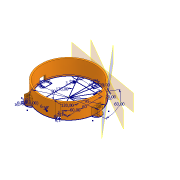
# Autodesk Inventor part: TopPart
Saved by Autodesk Inventor 2020.3 (Build 243373000, 373)
## iProperties
Created: 2021-08-28
Part Number: TopPart
Material: Generic
Document SubType Name: Modeling
Designer: Yusuf
Mass: 20.7363 g
Surface Area: 175.802 cm^2
Volume: 20.7363 cm^3
Density: 1 g/cm^3
Appearance: Orange
Author: Yusuf
Autodesk Inventor part; units mm, degrees
ref_plane "YZ Plane" through (0, 0, 0) normal (1, 0, 0) x (0, 1, 0)
ref_plane "XZ Plane" through (0, 0, 0) normal (0, 1, 0) x (-1, 0, 0)
ref_plane "XY Plane" through (0, 0, 0) normal (0, 0, 1) x (1, 0, 0)
sketch "Sketch1" plane through (0, 0, 0) normal (0, 1, 0) x (-1, 0, 0)
  circle A0 centre (0, 0) radius 47.5
  line L0 (0, 0) -> (23.75, 41.1362)
  line L1 (0, 0) -> (23.75, -41.1362)
  line L2 (0, 0) -> (-47.5, 0)
  circle A1 centre (23.75, 41.1362) radius 8
  circle A2 centre (25.75, 44.6003) radius 1.7
  circle A3 centre (25.75, 44.6003) radius 3.25
  line L3 (23.75, 41.1362) -> (27.75, 48.0644)
  arc A4 (30.4398, 45.5233) -> (30.3168, 36.567) centre (39.3185, 40.9223) ccw
  arc A5 (29.9181, 44.333) -> (29.4758, 46.7233) centre (27.662, 45.1516) ccw
  arc A6 (16.5096, 44.5386) -> (24.2044, 49.1233) centre (15.7805, 54.512) ccw
  arc A7 (25.7257, 48.8884) -> (23.4345, 48.0763) centre (25.2714, 46.5318) ccw
  circle A8 centre (-47.5, 0) radius 8
  arc A9 (-54.6442, 3.6) -> (-46.8263, 7.9716) centre (-55.099, 13.5897) ccw
  circle A10 centre (-51.5, 0) radius 3.25
  circle A11 centre (-51.5, 0) radius 1.7
  line L4 (-47.5, 0) -> (-55.5, 0)
  arc A12 (-53.3526, 3.7433) -> (-55.2014, 2.1651) centre (-52.9334, 1.3802) ccw
  arc A13 (-55.2014, -2.1651) -> (-53.3526, -3.7433) centre (-52.9334, -1.3802) ccw
  arc A14 (-46.8263, -7.9716) -> (-54.6442, -3.6) centre (-55.099, -13.5897) ccw
  circle A15 centre (23.75, -41.1362) radius 8
  arc A16 (24.2044, -49.1233) -> (16.5096, -44.5386) centre (15.7805, -54.512) ccw
  circle A17 centre (25.75, -44.6003) radius 3.25
  circle A18 centre (25.75, -44.6003) radius 1.7
  line L5 (23.75, -41.1362) -> (27.75, -48.0644)
  arc A19 (23.4345, -48.0763) -> (25.7257, -48.8884) centre (25.2714, -46.5318) ccw
  arc A20 (29.4758, -46.7233) -> (29.9181, -44.333) centre (27.662, -45.1516) ccw
  arc A21 (30.3168, -36.567) -> (30.4398, -45.5233) centre (39.3185, -40.9223) ccw
  line L6 (47.2466, -4.9) -> (47.2466, 4.9)
  line L7 (47.2466, 4.9) -> (35.2466, 4.9)
  line L8 (35.2466, 4.9) -> (35.2466, -4.9)
  line L9 (35.2466, -4.9) -> (47.2466, -4.9)
  line L10 (35.2466, -4.9) -> (41.2569, -4.9)
  line L11 (41.2569, -4.9) -> (41.2569, -6.9)
  line L12 (41.2569, -6.9) -> (35.2466, -6.9)
  line L13 (35.2466, -6.9) -> (35.2466, -4.9)
  line L14 (35.2466, 4.9) -> (41.2466, 4.9)
  line L15 (41.2466, 4.9) -> (41.2466, 6.9)
  line L16 (41.2466, 6.9) -> (35.2466, 6.9)
  line L17 (35.2466, 6.9) -> (35.2466, 4.9)
  line L18 (0, 0) -> (-23.75, 41.1362)
  line L19 (-26.3424, 39.5263) -> (-21.0596, 42.5763)
  line L20 (-21.0596, 42.5763) -> (-17.0596, 35.6481)
  line L21 (-17.0596, 35.6481) -> (-22.3424, 32.5981)
  line L22 (-22.3424, 32.5981) -> (-26.3424, 39.5263)
  line L23 (0, 0) -> (-23.75, -41.1362)
  line L24 (0, 0) -> (-36.3871, -30.5324)
  line L25 (0, 0) -> (-8.2483, -46.7784)
  line L26 (-28.9012, -20.6611) -> (-25.3659, -24.8744)
  line L27 (-25.3659, -24.8744) -> (-34.5584, -32.5878)
  line L28 (-28.9012, -20.6611) -> (-38.0937, -28.3746)
  line L29 (-20.0917, -29.2999) -> (-15.3286, -32.0499)
  line L30 (-15.3286, -32.0499) -> (-21.3286, -42.4422)
  line L31 (-20.0917, -29.2999) -> (-26.0917, -39.6922)
  line L32 (-8.8589, -34.4047) -> (-3.4425, -35.3597)
  line L33 (-3.4425, -35.3597) -> (-5.5262, -47.1774)
  line L34 (-8.8589, -34.4047) -> (-10.9427, -46.2224)
  line L35 (-38.0937, -28.3746) -> (-34.5584, -32.5878)
  line L36 (-26.0917, -39.6922) -> (-21.3286, -42.4422)
  line L37 (-10.9427, -46.2224) -> (-5.5262, -47.1774)
  line L38 (20, 30) -> (-20, 30)
  line L39 (-20, 30) -> (-20, -30)
  line L40 (-20, -30) -> (20, -30)
  line L41 (20, -30) -> (20, 30)
  circle A22 centre (17.4, -27.1) radius 1.6
  circle A23 centre (17.4, 27.1) radius 1.6
  circle A24 centre (-17.4, -27.1) radius 1.6
  circle A25 centre (-17.4, 27.1) radius 1.6
  circle A26 centre (0, 38) radius 1.5
  circle A27 centre (0, 38) radius 3
  circle A28 centre (0, 0) radius 45
  line L42 (0, 0) -> (0, -47.5)
  line L43 (-2, -43.4579) -> (2, -43.4579)
  line L44 (2, -43.4579) -> (2, -47.4579)
  line L45 (2, -47.4579) -> (-2, -47.4579)
  line L46 (-2, -47.4579) -> (-2, -43.4579)
  point P0 (-23.75, 0)
  point P1 (16.5096, 44.5386)
  point P2 (25.7257, 48.8884)
  point P3 (-46.8263, 7.9716)
  point P4 (-55.2014, -2.1651)
  point P5 (-46.8263, -7.9716)
  point P6 (29.4758, -46.7233)
  point P7 (30.3168, -36.567)
  point P8 (16.5096, -44.5386)
  point P9 (47.2466, 0)
  point P10 (-19.701, 34.1231)
  point P11 (-23.701, 41.0513)
  point P12 (-27.1335, -22.7677)
  point P13 (-17.7102, -30.6749)
  point P14 (-6.1507, -34.8822)
  point P15 (0, 30)
  point P16 (-20, 0)
  point P17 (-16.3362, 28.2951)
  point P18 (-15.8331, 27.4237)
  point P19 (47.2466, 4.9)
  point P20 (-19.8069, 40.4065)
  point P21 (-25.0896, 37.3565)
  point P22 (44.7324, 4.9)
  point P23 (44.7324, -4.9)
  point P24 (-20, -29.3529)
  point P25 (-18.8791, -30)
  point P26 (0, -43.4579)
  dimension "d0" = 95
  dimension "d1" = 120
  dimension "d2" = 120
  dimension "d3" = 16
  dimension "d4" = 3.4
  dimension "d5" = 6.5
  dimension "d7" = 10
  dimension "d8" = 3.6
  dimension "d9" = 2.4
  dimension "d10" = 1.2
  dimension "d15" = 360
  dimension "d17" = 9.8
  dimension "d18" = 12
  dimension "d19" = 2
  dimension "d20" = 6
  dimension "d21" = 2
  dimension "d23" = 60
  dimension "d24" = 6.1
  dimension "d25" = 8
  dimension "d26" = 6.1
  dimension "d27" = 60
  dimension "d28" = 20
  dimension "d29" = 20
  dimension "LedLength" = 5.5
  dimension "LedWidth" = 12
  dimension "d56" = 40
  dimension "d57" = 60
  dimension "d58" = 3.2
  dimension "d59" = 1.3
  dimension "d60" = 1
  dimension "d61" = 1
  dimension "d62" = 1.3
  dimension "d64" = 3
  dimension "d65" = 8
  dimension "d66" = 6
  dimension "d74" = 90
  dimension "d115" = 4
  dimension "d116" = 4
  constraints: 94 end point, 42 point on circle, 28 centre point, 15 perpendicular, 13 midpoint, 8 parallel, 7 coincident, 7 equal length, 6 symmetric about line, 5 horizontal alignment, 5 point on line, 4 horizontal, 4 vertical alignment, 3 equal radius, 2 vertical, 1 collinear, 1 tangent, 95 other
  measures "d1" angle of L1 L0
  measures "d2" angle of L2 L0
  measures "d3" diameter of A1
  measures "d4" diameter of A2
  measures "d5" diameter of A3
  measures "d7" radius of A4
  measures "d8" distance from line of L3 A1.end
  measures "d9" radius of A5
  measures "d10" vertical distance of A1.end A5.end
  measures "d17" distance of L6.start L6.end
  measures "d18" distance of L6.end L7.end
  measures "d19" distance of L10.end L11.end
  measures "d20" distance of L16.end L15.end
  measures "d21" distance of L15.end L14.end
  measures "d23" angle of L2 L18
  measures "d24" distance of L19.start L19.end
  measures "d25" distance of L19.end L20.end
  measures "d26" distance of L20.end L21.end
  measures "d27" angle of L2 L23
  measures "d28" angle of L24 L23
  measures "d29" angle of L25 L23
  measures "LedLength" distance of L32.start L32.end
  measures "LedWidth" distance of L32.end L33.end
  measures "d56" distance of L40.end L39.end
  measures "d57" distance of L39.end L38.end
  measures "d58" diameter of A22
  measures "d59" distance edge to line of A22 L40
  measures "d60" distance edge to line of A22 L41
  measures "d61" distance edge to line of A25 L39
  measures "d62" distance edge to line of A25 L38
  measures "d64" diameter of A26
  measures "d65" distance from line of L38 A26.centre
  measures "d66" diameter of A27
  measures "d74" diameter of A28
  measures "d115" distance of L44.end L45.end
  measures "d116" distance of L43.end L44.end
extrude "Extrusion9" add sketch "Sketch1" along normal blind 26 contours L7 A28 A1 A0 | L6 L9 A28 L7 | A0 A15 A28 L9 | A1 A28 L0 A0 | A0 L1 A28 A15 | L0 A28 A1 A0 | A0 A15 A28 L1 | A1 A28 L20 A0 | A0 L44 A28 A15 | L20 A28 L18 L19 | L45 L42 A28 L44 | A0 L42 L45 | L18 A28 L22 L19 | A0 L45 L42 | L45 L46 A28 L42 | L22 A28 A8 A0 | A0 L33 A28 L46 | A8 A28 L2 A0 | L37 L25 A28 L33 | A0 L25 L37 | L2 A28 A8 A0 | A0 L37 L25 | L37 L34 A28 L25 | A8 A28 L28 A0 | A0 L30 A28 L34 | A28 L30 L36 L23 | L23 L36 L31 A28 | A28 L27 L35 L24 | L24 L35 L28 A28 | L35 L24 A0 | A0 L23 L36 | L23 A0 L36 | L31 A0 L27 A28 | L35 A0 L24
extrude "Extrusion13" cut sketch "Sketch1" along normal blind 4.2 contours L20 A28 L18 L19 | L18 A28 L22 L19
extrude "Extrusion14" cut sketch "Sketch1" along normal blind 8.4 contours L6 L9 A28 L7
extrude "Extrusion16" add sketch "Sketch1" along normal blind 12.5 contours A0 L3 A3 A1 A5 A4 | A21 A20 A15 L5 A17 A0 | A0 A6 A7 A1 L3 A3 | L5 A17 A15 A19 A16 A0 | L3 A2 A3 | A3 L3 A2 | L5 A18 A17 | A17 L5 A18 | A0 L4 A10 A8 A12 A9 | A0 A14 A13 A8 L4 A10 | L4 A11 A10 | A10 L4 A11
sketch "Sketch8" plane through (0, 12.5, 0) normal (0, 1, 0) x (1, 0, 0)
  circle A0 centre (-25.75, -44.6003) radius 3.25
  circle A1 centre (-25.75, 44.6003) radius 1.7 projected
  circle A2 centre (-25.75, 44.6003) radius 3
  circle A3 centre (51.5, 0) radius 1.7 projected
  circle A4 centre (51.5, 0) radius 3
  point P0 (0, 0)
  dimension "d101" = 6.5
  dimension "d102" = 6
  dimension "d103" = 6
  constraints: 3 centre point, 3 coincident
  measures "d101" diameter of A0
  measures "d102" diameter of A2
  measures "d103" diameter of A4
extrude "Extrusion17" cut sketch "Sketch8" against normal blind 3
ref_plane "Work Plane5" through (38.0937, 0, -28.3746) normal (-0.7660444, 0, 0.6427876) x (-0.6427876, 0, -0.7660444)
ref_plane "Work Plane6" through (26.0917, 0, -39.6922) normal (-0.5, 0, 0.8660254) x (-0.8660254, 0, -0.5)
ref_plane "Work Plane7" through (10.9427, 0, -46.2224) normal (-0.1736482, 0, 0.9848078) x (-0.9848078, 0, -0.1736482)
sketch "Sketch12" plane through (38.0937, 0, -28.3746) normal (-0.7660444, 0, 0.6427876) x (-0.6427876, 0, -0.7660444)
  circle A0 centre (2.75, 0) radius 2.75
  point P0 (0, 0)
  point P1 (5.5, 0)
  dimension "d126" = 5.5
  constraints: 1 centre point, 1 coincident
  measures "d126" diameter of A0
sketch "Sketch13" plane through (26.0917, 0, -39.6922) normal (-0.5, 0, 0.8660254) x (-0.8660254, 0, -0.5)
  circle A0 centre (2.75, 0) radius 2.75
  dimension "d127" = 5.5
  constraints: 1 centre point, 1 coincident
  measures "d127" diameter of A0
sketch "Sketch14" plane through (10.9427, 0, -46.2224) normal (-0.1736482, 0, 0.9848078) x (-0.9848078, 0, -0.1736482)
  circle A0 centre (2.75, 0) radius 2.75
  dimension "d128" = 5.5
  constraints: 1 centre point, 1 coincident
  measures "d128" diameter of A0
extrude "Extrusion21" cut sketch "Sketch12" along normal mid plane 10
extrude "Extrusion22" cut sketch "Sketch13" against normal mid plane 10
extrude "Extrusion23" cut sketch "Sketch14" against normal mid plane 10
body "Solid2"
